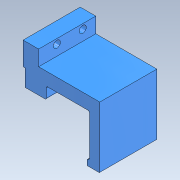
# Autodesk Inventor part: mount_bracket
Saved by Autodesk Inventor 2022.5 (Build 265521000, 521)
## iProperties
Created: 2022-05-25
Part Number: mount_bracket
Material: Generic
Document SubType Name: Modeling
Designer: SB13FLLT004
Density: 1 g/cm^3
Appearance: Cyan
Author: SB13FLLT004
Autodesk Inventor part; units mm, degrees
ref_plane "YZ Plane" through (0, 0, 0) normal (1, 0, 0) x (0, 1, 0)
ref_plane "XZ Plane" through (0, 0, 0) normal (0, 1, 0) x (-1, 0, 0)
ref_plane "XY Plane" through (0, 0, 0) normal (0, 0, 1) x (1, 0, 0)
derived "main_manifold_8v_v02.ipt"
sketch "Sketch:MM: main inlet" plane through (0, 0, 0) normal (1, 0, 0) x (0, 1, 0)
  line L0 (20.32, 0) -> (0, 0)
  line L1 (0, 0) -> (0, -27.94)
  line L2 (0, -27.94) -> (20.32, -27.94)
  line L3 (20.32, -27.94) -> (20.32, 0)
  point P0 (13.97, -15.24)
sketch "Sketch:MM: mounting screws:1" plane through (0, 0, 0) normal (-1, 0, 0) x (0, 0, 1)
  line L0 (-27.94, 0) -> (-27.94, 16.256)
  line L1 (-21.59, 5.08) -> (-8.89, 5.08) construction
  point P0 (0, 0)
  point P1 (-15.24, 13.97)
  point P2 (-15.24, 5.08)
sketch "Sketch: reference" plane through (0, 0, 0) normal (0, 0, 1) x (1, 0, 0)
  line L0 (-24.765, -0.4572) -> (-2.159, -0.4572)
  line L1 (-2.159, -0.4572) -> (-2.159, -4.2672)
  line L2 (-2.159, -4.2672) -> (-24.765, -4.2672)
  line L3 (-24.765, -4.2672) -> (-24.765, -0.4572)
  line L4 (-24.765, 20.32) -> (0, 20.32)
  line L5 (0, 0) -> (-24.765, 0)
  line L6 (-24.765, 0) -> (-24.765, 20.32)
  line L7 (0, 20.32) -> (0, 0) projected
  line L8 (-10.6362, -4.2672) -> (-10.6362, -8.8392)
  line L9 (-10.6362, -8.8392) -> (-1.016, -8.8392)
  line L10 (-1.016, -8.8392) -> (-1.016, -25.2984)
  dimension "d43" = 3.81
  dimension "d45" = 0.4572
  dimension "d47" = 22.606
  dimension "d48" = 2.159
  dimension "d49" = 4.572
  dimension "d50" = 1.016
  dimension "d51" = 8.4772
  constraints: 20 end point, 9 perpendicular, 1 coincident, 1 collinear, 1 point on line
  measures "d43" distance of L0.end L1.end
  measures "d45" distance between parallel lines of L0 L5
  measures "d47" distance of L1.end L2.end
  measures "d48" distance between parallel lines of L7 L1
  measures "d49" distance of L8.start L8.end
  measures "d50" distance between parallel lines of L10 L7
  measures "d51" distance between parallel lines of L8 L1
sketch "Sketch: side profile" plane through (0, 0, 0) normal (0, 0, 1) x (1, 0, 0)
  line L0 (11.93, -6.35) -> (31.93, -6.35) construction
  line L1 (31.93, -6.35) -> (31.93, -26.35) construction
  line L2 (31.93, -26.35) -> (11.93, -26.35) construction
  line L3 (11.93, -26.35) -> (11.93, -6.35) construction
  line L4 (11.43, -12.065) -> (1.016, -12.065)
  line L5 (1.016, -12.065) -> (1.016, 0)
  line L6 (1.016, 0) -> (37.51, 0)
  line L7 (37.51, 0) -> (37.51, -25.08)
  line L8 (37.51, -25.08) -> (32.43, -25.08)
  line L9 (32.43, -25.08) -> (32.43, -6.35)
  line L10 (32.43, -6.35) -> (11.43, -6.35)
  line L11 (11.43, -6.35) -> (11.43, -12.065)
  line L12 (11.43, -7.62) -> (11.93, -7.62) construction
  line L13 (32.43, -7.62) -> (31.93, -7.62) construction
  line L14 (0, -3.81) -> (0, 0)
  line L15 (0, 0) -> (1.016, 0)
  line L16 (1.016, -6.35) -> (11.43, -6.35)
  line L17 (31.414, -27.1) -> (37.51, -27.1)
  line L18 (37.51, -27.1) -> (37.51, -30.021)
  line L19 (37.51, -30.021) -> (31.414, -30.021)
  line L20 (31.414, -30.021) -> (31.414, -27.1)
  line L21 (37.51, -25.08) -> (37.51, -27.1)
  line L22 (32.43, -25.08) -> (32.43, -27.1)
  line L23 (0, -3.81) -> (1.016, -3.81)
  line L24 (0, 20.32) -> (0, 0) construction
  line L25 (-2.159, -4.2672) -> (-24.765, -4.2672) construction
  line L26 (-24.765, -0.4572) -> (-2.159, -0.4572) construction
  line L27 (-2.159, -0.4572) -> (-2.159, -4.2672) construction
  line L28 (-24.765, 20.32) -> (0, 20.32) construction
  line L29 (0, 0) -> (-24.765, 0) construction
  line L30 (-1.016, -8.8392) -> (-1.016, -25.2984) construction
  line L31 (-10.6362, -8.8392) -> (-1.016, -8.8392) construction
  line L32 (-10.6362, -4.2672) -> (-10.6362, -8.8392) construction
  line L33 (53.975, 22.4728) -> (53.975, 6.8361) construction
  point P0 (1.016, -5.08)
  point P1 (0, 0)
  point P2 (0, -3.8003)
  dimension "d1" = 20
  dimension "d2" = 0.5
  dimension "d3" = 6.35
  dimension "d4" = 5.08
  dimension "d16" = 1.27
  dimension "d22" = 1.016
  dimension "d26" = 0.75
  dimension "d27" = 1.016
  dimension "d28" = 2.921
  dimension "d30" = 1.27
  dimension "d34" = 11.93
  dimension "d52" = 3.81
  dimension "d53" = 53.975
  dimension "d56" = 12.065
  dimension "d57" = 21
  dimension "d58" = 10.414
  dimension "d59" = 11.43
  constraints: 50 end point, 19 perpendicular, 7 point on line, 4 horizontal, 3 collinear, 2 equal length, 1 parallel
  measures "d1" distance of L0.start L0.end
  measures "d2" distance of L13.start L13.end
  measures "d3" distance between parallel lines of L6 L10
  measures "d4" distance of L7.end L8.end
  measures "d16" distance between parallel lines of L2 L8
  measures "d22" distance between parallel lines of L14 L5
  measures "d26" distance between parallel lines of L17 L2
  measures "d27" distance between parallel lines of L20 L9
  measures "d28" distance of L19.end L17.start
  measures "d30" distance between parallel lines of L0 L13
  measures "d34" distance between parallel lines of L14 L3
  measures "d52" distance of L14.start L14.end
  measures "d53" distance between parallel lines of L33 L24
  measures "d56" distance between parallel lines of L4 L6
  measures "d57" distance between parallel lines of L11 L9
  measures "d58" distance of L4.start L4.end
  measures "d59" distance between parallel lines of L11 L14
sketch "Sketch: MM holes" plane through (0, 0, 0) normal (1, 0, 0) x (0, 1, 0)
  line L0 (20.32, -27.94) -> (20.32, 0) construction
  line L1 (20.32, 0) -> (0, 0) construction
  line L2 (0, -27.94) -> (20.32, -27.94) construction
  line L3 (0, 0) -> (0, -27.94) construction
  circle A0 centre (5.08, -8.89) radius 1.2065 construction
  line L4 (7.493, 0) -> (0, 0)
  line L5 (0, 0) -> (0, -27.94)
  line L6 (0, -27.94) -> (7.493, -27.94)
  line L7 (7.493, -27.94) -> (7.493, 0)
  point P0 (5.08, -21.59)
  dimension "d5" = 2.413
  dimension "d21" = 7.493
  constraints: 8 end point, 3 collinear, 3 perpendicular, 1 centre point, 1 coincident, 1 vertical
  measures "d5" diameter of A0
  measures "d21" distance of L5.end L6.end
extrude "Ex: MM screws" add sketch "Sketch: MM holes" along normal blind 7.62
hole "Hole: MM screws (4-40)" at (0, 5.08, -8.89) at (0, 5.08, -21.59) direction (1, 0, 0) diameter 3.429 end through all
extrude "Ex: side profile" add sketch "Sketch: side profile" against normal up to surface (27.94 mm away) from surface at 0
fillet "Fillet1" radius 0.635 4 edges at (11.43, -6.35, -13.97) (32.43, -6.35, -13.97) (11.43, -12.065, -13.97) (32.43, -27.1, -13.97)
fillet "Fillet2" radius 0.254 3 edges at (31.414, -30.021, -13.97) (37.51, -30.021, -13.97) (31.414, -27.1, -13.97)
body "Solid1"
